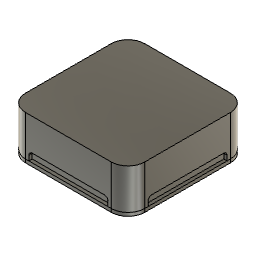
soap_case (Autodesk Fusion 360 design; units mm, degrees)
Autodesk Fusion 360 part; units mm, degrees
sketch "Sketch1" plane through (0, 0, 0) normal (0, 0, 1) x (1, 0, 0)
  line L0 (-9, 15) -> (42, 15)
  line L1 (48, 9) -> (48, -42)
  line L2 (42, -48) -> (-9, -48)
  line L3 (-15, -42) -> (-15, 9)
  arc A0 (-9, 15) -> (-15, 9) centre (-9, 9) ccw
  arc A1 (48, 9) -> (42, 15) centre (42, 9) ccw
  arc A2 (42, -48) -> (48, -42) centre (42, -42) ccw
  arc A3 (-15, -42) -> (-9, -48) centre (-9, -42) ccw
  arc A4 (-9, 17) -> (-17, 9) centre (-9, 9) ccw
  line L4 (-17, -42) -> (-17, 9)
  arc A5 (-17, -42) -> (-9, -50) centre (-9, -42) ccw
  line L5 (42, -50) -> (-9, -50)
  arc A6 (42, -50) -> (50, -42) centre (42, -42) ccw
  line L6 (50, 9) -> (50, -42)
  arc A7 (50, 9) -> (42, 17) centre (42, 9) ccw
  line L7 (-9, 17) -> (42, 17)
  arc A8 (-9, 19) -> (-19, 9) centre (-9, 9) ccw
  line L8 (-19, -42) -> (-19, 9)
  arc A9 (-19, -42) -> (-9, -52) centre (-9, -42) ccw
  line L9 (42, -52) -> (-9, -52)
  arc A10 (42, -52) -> (52, -42) centre (42, -42) ccw
  line L10 (52, 9) -> (52, -42)
  arc A11 (52, 9) -> (42, 19) centre (42, 9) ccw
  line L11 (-9, 19) -> (42, 19)
  arc A12 (50.2, 9) -> (42, 17.2) centre (42, 9) ccw
  line L12 (-9, 17.2) -> (42, 17.2)
  arc A13 (-9, 17.2) -> (-17.2, 9) centre (-9, 9) ccw
  line L13 (-17.2, -42) -> (-17.2, 9)
  arc A14 (-17.2, -42) -> (-9, -50.2) centre (-9, -42) ccw
  line L14 (42, -50.2) -> (-9, -50.2)
  arc A15 (42, -50.2) -> (50.2, -42) centre (42, -42) ccw
  line L15 (50.2, 9) -> (50.2, -42)
  point P0 (-15, 15)
  point P1 (48, 15)
  point P2 (-15, -48)
  dimension "d1" = 63
  dimension "d2" = 63
  dimension "d3" = 6
  dimension "d4" = -2
  dimension "d5" = -4
  dimension "d10" = -2.2
  constraint horizontal L0
  constraint vertical L1
  constraint horizontal L2
  constraint vertical L3
  constraint coincident P0 L0
  constraint coincident P0 L3
  constraint tangent L0 A0
  constraint tangent L3 A0
  constraint coincident P1 L0
  constraint coincident P1 L1
  constraint tangent L0 A1
  constraint tangent L1 A1
  constraint equal A0 A1
  constraint tangent L1 A2
  constraint tangent L2 A2
  constraint equal A0 A2
  constraint coincident P2 L2
  constraint coincident P2 L3
  constraint tangent L2 A3
  constraint tangent L3 A3
  constraint equal A0 A3
  measures "d1" distance of P0 P1
  measures "d2" distance of P0 P2
  measures "d3" radius of A0
extrude "Extrude1" add sketch "Sketch1" along normal blind 8 contours A4 L4 A5 L5 A6 L6 A7 L7 makes body 1
extrude "Extrude2" add sketch "Sketch1" against normal blind 2 contours L0 L1 L2 L3 A0 A1 A2 A3 | A4 L4 A5 L5 A6 L6 A7 L7 | A8 L8 A9 L9 A10 L10 A11 L11 | A12 L12 A13 L13 A14 L14 A15 L15 bodies 1
extrude "Extrude1'" add sketch "Sketch1" along normal blind 22 separate body contours A8 L8 A9 L9 A10 L10 A11 L11 makes body 2 in component "Component"
sketch "Sketch2" plane through (0, 0, 22) normal (0, 0, 1) x (-1, 0, 0)
  arc A0 (9, -17.2) -> (17.2, -9) centre (9, -9) ccw
  line L0 (9, -17.2) -> (-42, -17.2)
  arc A1 (-50.2, -9) -> (-42, -17.2) centre (-42, -9) ccw
  line L1 (-50.2, -9) -> (-50.2, 42)
  arc A2 (-42, 50.2) -> (-50.2, 42) centre (-42, 42) ccw
  line L2 (-42, 50.2) -> (9, 50.2)
  arc A3 (17.2, 42) -> (9, 50.2) centre (9, 42) ccw
  line L3 (17.2, 42) -> (17.2, -9)
  arc A4 (19, 42) -> (9, 52) centre (9, 42) ccw
  line L4 (9, 52) -> (-42, 52)
  arc A5 (-42, 52) -> (-52, 42) centre (-42, 42) ccw
  line L5 (-52, 42) -> (-52, -9)
  arc A6 (-52, -9) -> (-42, -19) centre (-42, -9) ccw
  line L6 (-42, -19) -> (9, -19)
  arc A7 (9, -19) -> (19, -9) centre (9, -9) ccw
  line L7 (19, -9) -> (19, 42)
  line L8 (-24.5335, -19) -> (25, -19) construction
  line L9 (19, -5.9098) -> (19, -23.1941) construction
  line L10 (-52, 36.1857) -> (-52, 61.8333) construction
  line L11 (-39.3087, 52) -> (-56.3142, 52) construction
  line L12 (9, -19) -> (-42, -19)
  line L13 (-52, -9) -> (-52, 42)
  line L14 (-42, 52) -> (9, 52)
  line L15 (19, 42) -> (19, -9)
  arc A8 (9, -19) -> (19, -9) centre (9, -9) ccw
  arc A9 (-52, -9) -> (-42, -19) centre (-42, -9) ccw
  arc A10 (-42, 52) -> (-52, 42) centre (-42, 42) ccw
  arc A11 (19, 42) -> (9, 52) centre (9, 42) ccw
  dimension "d13" = 10
  constraint coincident L6 L8.start
  constraint coincident L7 L9.start
  constraint perpendicular L8 L9
  constraint coincident L5 L10.start
  constraint parallel L5 L10
  constraint coincident L4 L11.start
  constraint perpendicular L10 L11
  constraint horizontal L12
  constraint vertical L13
  constraint horizontal L14
  constraint vertical L15
  constraint tangent L12 A8
  constraint tangent L15 A8
  constraint tangent L12 A9
  constraint tangent L13 A9
  constraint equal A8 A9
  constraint tangent L13 A10
  constraint tangent L14 A10
  constraint equal A8 A10
  constraint tangent L14 A11
  constraint tangent L15 A11
  constraint equal A8 A11
  measures "d13" radius of A8
extrude "Extrude2'" add sketch "Sketch2" along normal blind 2 contours A0 L0 A1 L1 A2 L2 A3 L3 | A4 L4 A5 L5 A6 L6 A7 L7 L12 L13 L14 L15 A8 A9 A10 A11 bodies 2 in component "Component"
sketch "Sketch3" plane through (52, 0, 0) normal (1, 0, 0) x (0, 1, 0)
  line L0 (-42, 0) -> (9, 0)
  line L1 (9, 0) -> (9, 24)
  line L2 (9, 24) -> (-42, 24)
  line L3 (-42, 24) -> (-42, 0)
  line L4 (-40, 0) -> (7, 0)
  line L5 (7, 0) -> (7, 3)
  line L6 (5, 5) -> (-38, 5)
  line L7 (-40, 3) -> (-40, 0)
  arc A0 (-38, 5) -> (-40, 3) centre (-38, 3) ccw
  arc A1 (7, 3) -> (5, 5) centre (5, 3) ccw
  dimension "d16" = 2
  constraint horizontal L4
  constraint vertical L5
  constraint horizontal L6
  constraint vertical L7
  constraint coincident L0 L4.start
  constraint tangent L6 A0
  constraint tangent L7 A0
  constraint tangent L5 A1
  constraint tangent L6 A1
  constraint equal A0 A1
  measures "d16" radius of A0
extrude "Extrude3" cut sketch "Sketch3" against normal blind 2 contours L0 L4 L5 L6 L7 A0 A1 bodies 2 in component "Component"
sketch "Sketch4" plane through (0, -52, 0) normal (0, -1, 0) x (1, 0, 0)
  line L0 (-9, 0) -> (42, 0)
  line L1 (42, 0) -> (42, 24)
  line L2 (42, 24) -> (-9, 24)
  line L3 (-9, 24) -> (-9, 0)
  line L4 (-7, 0) -> (40, 0)
  line L5 (40, 0) -> (40, 3)
  line L6 (38, 5) -> (-5, 5)
  line L7 (-7, 3) -> (-7, 0)
  arc A0 (-5, 5) -> (-7, 3) centre (-5, 3) ccw
  arc A1 (40, 3) -> (38, 5) centre (38, 3) ccw
  dimension "d19" = 2
  constraint horizontal L4
  constraint vertical L5
  constraint horizontal L6
  constraint vertical L7
  constraint coincident L0 L4.start
  constraint tangent L6 A0
  constraint tangent L7 A0
  constraint tangent L5 A1
  constraint tangent L6 A1
  constraint equal A0 A1
  measures "d19" radius of A0
extrude "Extrude4" cut sketch "Sketch4" against normal blind 2 contours L0 L4 L5 L6 L7 A0 A1 bodies 2 in component "Component"
sketch "Sketch5" plane through (0, 19, 0) normal (0, 1, 0) x (-1, 0, 0)
  line L0 (-42, 0) -> (9, 0)
  line L1 (9, 0) -> (9, 24)
  line L2 (9, 24) -> (-42, 24)
  line L3 (-42, 24) -> (-42, 0)
  line L4 (-40, 0) -> (7, 0)
  line L5 (7, 0) -> (7, 3)
  line L6 (5, 5) -> (-38, 5)
  line L7 (-40, 3) -> (-40, 0)
  arc A0 (-38, 5) -> (-40, 3) centre (-38, 3) ccw
  arc A1 (7, 3) -> (5, 5) centre (5, 3) ccw
  dimension "d22" = 2
  constraint horizontal L4
  constraint vertical L5
  constraint horizontal L6
  constraint vertical L7
  constraint coincident L0 L4.start
  constraint tangent L6 A0
  constraint tangent L7 A0
  constraint tangent L5 A1
  constraint tangent L6 A1
  constraint equal A0 A1
  measures "d22" radius of A0
extrude "Extrude5" cut sketch "Sketch5" against normal blind 2 contours L0 L4 L5 L6 L7 A0 A1 bodies 2 in component "Component"
sketch "Sketch6" plane through (-19, 0, 0) normal (-1, 0, 0) x (0, -1, 0)
  line L0 (-9, 0) -> (42, 0)
  line L1 (42, 0) -> (42, 24)
  line L2 (42, 24) -> (-9, 24)
  line L3 (-9, 24) -> (-9, 0)
  line L4 (-7, 0) -> (40, 0)
  line L5 (40, 0) -> (40, 3)
  line L6 (38, 5) -> (-5, 5)
  line L7 (-7, 3) -> (-7, 0)
  arc A0 (-5, 5) -> (-7, 3) centre (-5, 3) ccw
  arc A1 (40, 3) -> (38, 5) centre (38, 3) ccw
  dimension "d25" = 47
  dimension "d26" = 2
  constraint horizontal L4
  constraint vertical L5
  constraint horizontal L6
  constraint vertical L7
  constraint coincident L0 L4.start
  constraint tangent L6 A0
  constraint tangent L7 A0
  constraint tangent L5 A1
  constraint tangent L6 A1
  constraint equal A0 A1
  measures "d25" distance of L4.start L4.end
  measures "d26" radius of A0
extrude "Extrude6" cut sketch "Sketch6" against normal blind 2 contours L0 L4 L5 L6 L7 A0 A1 bodies 2 in component "Component"
component "Component" placed x (1, 0, 0) y (0, 1, 0) z (0, 0, 1) at (0, 0, 0)
